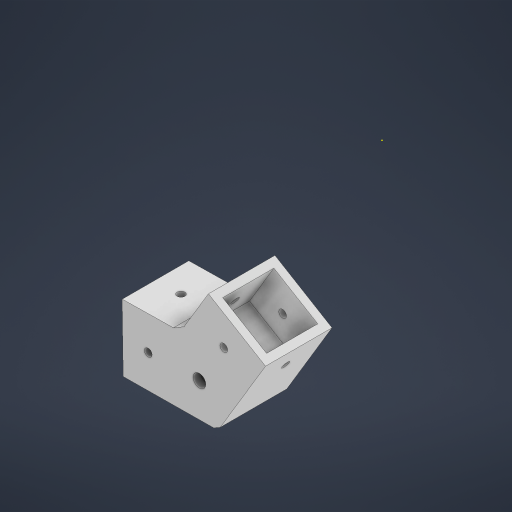
# Autodesk Inventor part: 2020_nodes_conn
Saved by Autodesk Inventor 2024 (Build 280153000, 153)
## iProperties
Created: 2026-03-28
Part Number: 2020_nodes_conn
Material: PET Plastic
Document SubType Name: Modeling
Designer: schar
Density: 1.541 g/cm^3
Appearance: Polycarbonate - Clear
Author: schar
Autodesk Inventor part; units mm, degrees
ref_plane "YZ Plane" through (0, 0, 0) normal (1, 0, 0) x (0, 1, 0)
ref_plane "XZ Plane" through (0, 0, 0) normal (0, 1, 0) x (-1, 0, 0)
ref_plane "XY Plane" through (0, 0, 0) normal (0, 0, 1) x (1, 0, 0)
sketch "Sketch1" plane through (0, 0, 0) normal (0, 0, 1) x (1, 0, 0)
  circle A0 centre (-48.3826, -94.0192) radius 2.5
  circle A1 centre (2.8152, 8.6005) radius 2.5
  line L0 (-48.3826, -94.0192) -> (40.5013, 54.4144)
  line L1 (2.8152, 8.6005) -> (32.8522, -42.034)
  line L2 (-2.0828, 38.9998) -> (-2.0828, -39)
  line L3 (-2.0828, -0.0001) -> (69.8745, -0.0001)
  line L4 (7.9172, -0.0001) -> (-0.6834, -5.1021)
  line L5 (2.8152, 8.6005) -> (7.9172, -0.0001)
  line L6 (7.9172, -0.0001) -> (16.5177, 5.1019)
  line L7 (7.9172, -0.0001) -> (-0.6834, -5.1021)
  line L8 (-0.6834, -5.1021) -> (-0.6834, -5.1021)
  line L9 (7.9172, -0.0001) -> (16.5177, 5.1019)
  line L10 (16.5177, 5.1019) -> (16.5177, 5.1019)
  line L11 (7.9172, -0.0001) -> (-0.6622, 5.1374)
  line L12 (7.9172, -0.0001) -> (16.4966, -5.1375)
  line L13 (-48.3826, -94.0192) -> (-43.2452, -85.4397)
  line L14 (-54.6233, -56.9895) -> (-9.7188, -83.8789)
  line L15 (-43.2452, -85.4397) -> (-34.6657, -90.5772)
  line L16 (-43.2452, -85.4397) -> (-51.8246, -80.3023)
  line L17 (-34.6657, -90.5772) -> (16.4966, -5.1375)
  line L18 (-0.6622, 5.1374) -> (-51.8246, -80.3023)
  line L19 (-3.7386, 0) -> (13.452, 10.2217)
  line L20 (-3.7386, 0) -> (13.4203, -10.2749)
  circle A2 centre (6.9172, -34) radius 2.5
  circle A3 centre (6.9172, -34) radius 5
  circle A4 centre (6.9172, 34) radius 2.5
  circle A5 centre (6.9172, 34) radius 4.9998
  line L21 (15.8878, 38.9998) -> (-2.0828, 38.9998)
  line L22 (-2.0828, -39) -> (15.933, -39)
  line L23 (-13.3434, -16.0398) -> (19.6624, -35.8041)
  line L24 (-13.3434, 16.0396) -> (19.6624, 35.8039)
  line L25 (-13.3434, -16.0398) -> (-15.9172, -14.4985)
  line L26 (-2.0828, -0.0001) -> (-26.2435, -0.0001)
  line L27 (-15.9172, -14.4985) -> (-7.2354, -0.0001)
  line L28 (-13.3434, 16.0396) -> (-15.9172, 14.4984)
  line L29 (-15.9172, 14.4984) -> (-7.2354, -0.0001)
  line L30 (13.4203, -10.2749) -> (15.9172, -11.7701)
  line L31 (15.933, -39) -> (15.8878, 38.9998)
  line L32 (13.452, 10.2217) -> (15.9037, 11.6795)
  line L33 (15.9037, 11.6795) -> (6.3124, 27.8097)
  line L34 (15.9172, -11.7701) -> (6.3124, -27.8099)
  line L35 (15.9037, 11.6795) -> (15.9172, -11.7701)
  line L36 (-15.9172, -14.4985) -> (-15.9172, 14.4984)
  line L37 (6.3124, 27.8097) -> (-15.9172, 14.4984) projected
  circle A6 centre (-48.3826, -94.0192) radius 2.5
  line L38 (-311.4249, 0) -> (127.5863, 0)
  line L39 (-170.3704, -117.2696) -> (-13.4682, 154.4931)
  line L40 (-102.6648, 0) -> (-157.9558, -95.7668)
  line L41 (-157.9558, -95.7668) -> (-48.3826, -94.0192)
  line L42 (-48.3826, -94.0192) -> (-58.3814, -94.1786)
  line L43 (-58.3814, -94.1786) -> (-58.5408, -84.1799)
  line L44 (-58.5408, -84.1799) -> (-58.2219, -104.1774)
  line L45 (-51.8246, -80.3023) -> (-41.5497, -63.1434)
  line L46 (-41.5497, -63.1434) -> (-24.3908, -73.4184)
  line L47 (-58.5408, -84.1799) -> (-78.5383, -84.4989)
  line L48 (-78.5383, -84.4989) -> (-78.2193, -104.4963)
  line L49 (-78.2193, -104.4963) -> (-58.2219, -104.1774)
  line L50 (-58.5408, -84.1799) -> (-51.8246, -80.3023)
  line L51 (-58.2219, -104.1774) -> (-26.2433, -104.1774)
  line L52 (-34.6657, -90.5772) -> (-48.6317, -113.8999)
  circle A7 centre (-48.3828, -94.0194) radius 2.5 projected
  point P0 (0, 0)
  point P1 (6.9172, -21)
  point P2 (-3.7386, 0)
  point P3 (-42.2878, -64.3761)
  point P4 (-42.8097, -104.1774)
  point P5 (-25.129, -74.6511)
  dimension "d0" = 10
  dimension "d1" = 10
  dimension "d2" = 10
  dimension "d3" = 10
  dimension "d4" = 10
  dimension "d5" = 10
  dimension "d6" = 10
  dimension "d7" = 10
  dimension "d8" = 10
  dimension "d9" = 10
  dimension "d10" = 10
  dimension "d11" = 20
  dimension "d12" = 20
  dimension "d13" = 3
  dimension "d14" = 3
  dimension "d20" = 110.582
  dimension "d21" = 10
  dimension "d22" = 10
  dimension "d23" = 20
  dimension "d24" = 20
  dimension "d25" = 20
  dimension "d26" = 121.827
  dimension "d27" = 146.9972
  constraints: 102 end point, 19 point on line, 17 perpendicular, 7 centre point, 5 collinear, 5 parallel, 3 coincident, 3 horizontal, 3 tangent, 2 equal radius, 2 midpoint, 2 symmetric about line, 10 other
  measures "d0" distance of L26.start L4.start
  measures "d1" distance of L4.start L4.end
  measures "d2" distance of L1.start L5.end
  measures "d3" distance of L5.end L6.end
  measures "d4" distance of L5.end L7.end
  measures "d5" distance of L4.start L9.end
  measures "d6" distance of L4.start L11.end
  measures "d7" distance of L4.start L12.end
  measures "d8" distance of L13.start L13.end
  measures "d9" distance of L13.end L15.end
  measures "d10" distance of L13.end L18.end
  measures "d11" distance of L20.start L19.end
  measures "d12" distance of L20.start L30.start
  measures "d13" distance of L25.start L25.end
  measures "d14" distance of L28.start L36.end
  measures "d20" distance of L40.start L40.end
  measures "d21" distance of L13.start L42.end
  measures "d22" distance of L42.end L43.end
  measures "d23" distance of L43.end L44.end
  measures "d24" distance of L18.end L45.end
  measures "d25" distance of L43.end L47.end
  measures "d26" angle of L42 L0
  measures "d27" distance from line of L0.end L42
extrude "Extrusion1" add sketch "Sketch1" against normal blind 3 contours A0 L0 L15 L52 L51 L44 L41 | A0 L41 L43 L50 L16 L0 | L16 L18 L14 L0 | L0 L14 L17 L15 | L44 L49 L48 L41 | L41 L48 L47 L43
sketch "Sketch2" plane through (0, 0, -3) normal (0, 0, -1) x (-1, 0, 0)
  line L0 (51.8246, -80.3023) -> (42.2878, -64.3761) projected
  line L1 (25.129, -74.6511) -> (42.8097, -104.1774) projected
  line L2 (78.5383, -84.4989) -> (58.5408, -84.1799)
  line L3 (58.5408, -84.1799) -> (51.8246, -80.3023)
  line L4 (42.2878, -64.3761) -> (25.129, -74.6511)
  line L5 (78.5383, -84.4989) -> (78.2193, -104.4963)
  line L6 (58.5408, -84.1799) -> (58.5408, -81.1799)
  line L7 (51.8246, -80.3023) -> (54.3984, -78.761)
  line L8 (42.8097, -104.1774) -> (40.2359, -105.7186)
  line L9 (42.8097, -104.1774) -> (42.7827, -107.1772)
  line L10 (78.5383, -84.4989) -> (78.5383, -81.4989)
  line L11 (78.2193, -104.4963) -> (78.2193, -107.4963)
  line L12 (42.2878, -64.3761) -> (44.8616, -62.8349)
  line L13 (42.2878, -64.3761) -> (25.129, -74.6511) projected
  line L14 (25.129, -74.6511) -> (22.5551, -76.1923)
  line L15 (78.5383, -81.4989) -> (58.5408, -81.1799)
  line L16 (58.5408, -81.1799) -> (54.3984, -78.761)
  line L17 (54.3984, -78.761) -> (44.8616, -62.8349)
  line L18 (22.5551, -76.1923) -> (40.2359, -105.7186)
  line L19 (40.2359, -105.7186) -> (42.7827, -107.1772)
  line L20 (78.2193, -107.4963) -> (42.7827, -107.1772)
  line L21 (58.5408, -84.1799) -> (58.2219, -104.1774)
  line L22 (51.8246, -80.3023) -> (34.6657, -90.5772)
  circle A0 centre (48.3826, -94.0192) radius 2.5 projected
  circle A1 centre (48.3826, -94.0192) radius 2.5
  line L23 (78.2193, -104.4963) -> (42.8097, -104.1774)
  line L24 (58.2219, -104.1774) -> (42.8097, -104.1774) projected
  line L25 (78.2193, -104.4963) -> (58.2219, -104.1774) projected
  point P0 (0, 0)
  dimension "d30" = 3
  dimension "d31" = 3
  dimension "d32" = 3
  dimension "d33" = 3
  dimension "d34" = 3
  dimension "d35" = 3
  dimension "d36" = 3
  dimension "d37" = 3
  constraints: 42 end point, 3 perpendicular, 3 vertical, 2 coincident, 2 collinear, 1 centre point, 1 point on line
  measures "d30" distance of L2.end L6.end
  measures "d31" distance of L0.start L7.end
  measures "d32" distance of L1.end L8.end
  measures "d33" distance of L1.end L9.end
  measures "d34" distance of L2.start L10.end
  measures "d35" distance of L5.end L11.end
  measures "d36" distance of L4.start L12.end
  measures "d37" distance of L1.start L14.end
extrude "Extrusion2" add sketch "Sketch2" along normal blind 20 and the other way blind 3 contours L7 L16 L6 L3 | L0 L12 L17 L7 | L6 L15 L10 L2 | L1 L8 L18 L14 | L25 L23 L24 | L9 L19 L8 | L23 L11 L20 L9
sketch "Sketch3" plane through (0, 0, -3) normal (0, 0, -1) x (-1, 0, 0)
  line L0 (58.5408, -84.1799) -> (51.8246, -80.3023) projected
  line L1 (51.8246, -80.3023) -> (34.6657, -90.5772)
  line L2 (25.129, -74.6511) -> (42.8097, -104.1774) projected
  line L3 (42.8097, -104.1774) -> (58.2219, -104.1774) projected
  line L4 (58.5408, -84.1799) -> (58.2219, -104.1774)
  line L5 (78.2193, -104.4963) -> (42.8097, -104.1774) projected
  line L6 (42.8097, -104.1774) -> (25.129, -74.6511) projected
  circle A0 centre (48.3828, -94.0194) radius 2.5 projected
  point P0 (0, 0)
  dimension "d42" = 119.086
  constraints: 4 end point, 1 coincident, 1 point on line
  measures "d42" angle of L1 L0
extrude "Extrusion3" add sketch "Sketch3" along normal blind 20
sketch "Sketch4" plane through (0, 0, -23) normal (0, 0, -1) x (-1, 0, 0)
  point P0 (0, 0)
sketch "Sketch5" plane through (0, 0, -23) normal (0, 0, -1) x (-1, 0, 0)
  circle A0 centre (48.3828, -94.0194) radius 2.5 projected
  line L0 (44.8616, -62.8349) -> (42.2878, -64.3761) projected
  line L1 (42.2878, -64.3761) -> (51.8246, -80.3023) projected
  line L2 (51.8246, -80.3023) -> (34.6657, -90.5772) projected
  line L3 (34.6657, -90.5772) -> (25.129, -74.6511) projected
  line L4 (25.129, -74.6511) -> (22.5551, -76.1923) projected
  line L5 (22.5551, -76.1923) -> (40.2359, -105.7186) projected
  line L6 (40.2359, -105.7186) -> (42.7827, -107.1772) projected
  line L7 (42.7827, -107.1772) -> (78.2193, -107.4963) projected
  line L8 (78.2193, -107.4963) -> (78.2193, -104.4963) projected
  line L9 (78.2193, -104.4963) -> (58.2219, -104.1774) projected
  line L10 (58.2219, -104.1774) -> (58.5408, -84.1799) projected
  line L11 (58.5408, -84.1799) -> (78.5383, -84.4989) projected
  line L12 (78.5383, -84.4989) -> (78.5383, -81.4989) projected
  line L13 (78.5383, -81.4989) -> (58.5408, -81.1799) projected
  line L14 (58.5408, -81.1799) -> (54.3984, -78.761) projected
  line L15 (54.3984, -78.761) -> (44.8616, -62.8349) projected
  line L16 (58.5408, -84.1799) -> (58.2219, -104.1774) projected
  line L17 (58.2219, -104.1774) -> (78.2193, -104.4963) projected
  line L18 (78.2193, -104.4963) -> (78.5383, -84.4989) projected
  line L19 (78.5383, -84.4989) -> (58.5408, -84.1799) projected
  line L20 (34.6657, -90.5772) -> (51.8246, -80.3023) projected
  line L21 (51.8246, -80.3023) -> (42.2878, -64.3761) projected
  line L22 (42.2878, -64.3761) -> (25.129, -74.6511) projected
  line L23 (25.129, -74.6511) -> (34.6657, -90.5772) projected
  point P0 (0, 0)
extrude "Extrusion4" add sketch "Sketch5" along normal blind 3
sketch "Sketch6" plane through (0, 0, 0) normal (0, 0, 1) x (1, 0, 0)
  line L0 (-42.2878, -64.3761) -> (-25.129, -74.6511) projected
  line L1 (-33.7084, -69.5136) -> (-49.5228, -95.9232)
  line L2 (-33.7084, -69.5136) -> (-38.8459, -78.093)
  circle A0 centre (-38.8459, -78.093) radius 1.5
  line L3 (-78.5383, -84.4989) -> (-78.2193, -104.4963) projected
  line L4 (-78.3788, -94.4976) -> (-68.3788, -94.4976)
  circle A1 centre (-68.3788, -94.4976) radius 1.5
  point P0 (0, 0)
  dimension "d47" = 10
  dimension "d48" = 3
  dimension "d56" = 10
  dimension "d57" = 3
  constraints: 6 end point, 2 centre point, 2 coincident, 2 midpoint, 1 horizontal, 1 perpendicular, 1 point on line
  measures "d47" distance of L1.start L2.end
  measures "d48" diameter of A0
  measures "d56" distance of L4.start L4.end
  measures "d57" diameter of A1
extrude "Extrusion5" cut sketch "Sketch6" against normal through all
sketch "Sketch7" plane through (-44.8616, -62.8349, -26) normal (-0.857942, 0.5137465, 0) x (0, 0, 1)
  line L0 (0, 0) -> (26, 0) projected
  line L1 (26, 0) -> (13, 0)
  line L2 (13, 0) -> (13, -10)
  line L3 (13, -10) -> (26, -10)
  line L4 (26, -10) -> (26, 0)
  circle A0 centre (13, -10) radius 1.5
  point P0 (26, 76.9562)
  dimension "d51" = 13
  dimension "d52" = 10
  dimension "d53" = 3
  constraints: 8 end point, 2 parallel, 1 centre point, 1 coincident, 1 horizontal, 1 perpendicular
  measures "d51" distance of L3.end L2.end
  measures "d52" distance of L2.end L1.end
  measures "d53" diameter of A0
extrude "Extrusion6" cut sketch "Sketch7" against normal through all contours A0 L3 L2 | L2 L3 A0
sketch "Sketch8" plane through (-58.5408, -81.1799, 0) normal (-0.0159478, 0.9998728, 0) x (0.9998728, 0.0159478, 0)
  line L0 (-20.0478, 3) -> (-20.0478, 23) projected
  line L1 (-20.0478, 13) -> (-10.0478, 13)
  circle A0 centre (-10.0478, 13) radius 1.5
  point P0 (59.828, 0)
  dimension "d58" = 10
  dimension "d59" = 3
  constraints: 2 end point, 1 centre point, 1 coincident, 1 horizontal, 1 midpoint
  measures "d58" distance of L1.start L1.end
  measures "d59" diameter of A0
extrude "Extrusion7" cut sketch "Sketch8" against normal through all
body "Solid1"
